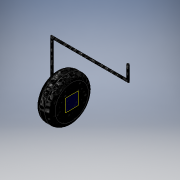
# Autodesk Inventor part: Main Landing Gear
Saved by Autodesk Inventor 2018 (Build 220112000, 112)
## iProperties
Created: 2018-08-04
Part Number: Main Landing Gear
Material: Generic
Document SubType Name: Modeling
Designer: Michael Gunderman
Density: 0.711196 g/cm^3
Appearance: Default
Mass: 81 g
Surface Area: 163.949 cm^2
Volume: 113.893 cm^3
Author: Michael Gunderman
Autodesk Inventor part; units mm, degrees
ref_plane "YZ Plane" through (0, 0, 0) normal (1, 0, 0) x (0, 1, 0)
ref_plane "XZ Plane" through (0, 0, 0) normal (0, 1, 0) x (-1, 0, 0)
ref_plane "XY Plane" through (0, 0, 0) normal (0, 0, 1) x (1, 0, 0)
ref_plane "Work Plane1" through (-36.0844, -34.5379, 0) normal (-1, 0, 0) x (0, -1, 0)
sketch "Sketch1" plane through (-36.0844, -34.5379, 0) normal (-1, 0, 0) x (0, -1, 0)
  circle A0 centre (0, 0) radius 37.75
  point P0 (-34.5379, 0)
  dimension "d4" = 75.5
  constraints: 1 centre point, 1 coincident
  measures "d4" diameter of A0
extrude "Extrusion1" add sketch "Sketch1" along normal blind 26.5
fillet "Fillet1" radius 9 2 edges at (-62.5844, 3.2121, 0) (-36.0844, 3.2121, 0)
sketch "Sketch2" plane through (-36.0844, -34.5379, 0) normal (-1, 0, 0) x (0, -1, 0)
  circle A0 centre (0, 0) radius 2
  point P0 (-34.5379, 0)
  dimension "d8" = 4
  constraints: 1 centre point
  measures "d8" diameter of A0
sketch3d "3D Sketch1"
  line L0 (-36.0844, -34.5379, 0) -> (-70.0844, -34.5379, 0)
  line L1 (-70.0844, -34.5379, 0) -> (-70.0844, 45.4621, 0)
  line L2 (-70.0844, 45.4621, 0) -> (60.9156, 45.4621, 0)
  line L3 (60.9156, 45.4621, 0) -> (60.9156, 70.4621, 0)
  dimension "d0" = 34
  dimension "d1" = 80
  dimension "d2" = 131
  dimension "d3" = 25
sweep "Sweep1" add profiles "Sketch2" path "3D Sketch1"
body "Solid1"
